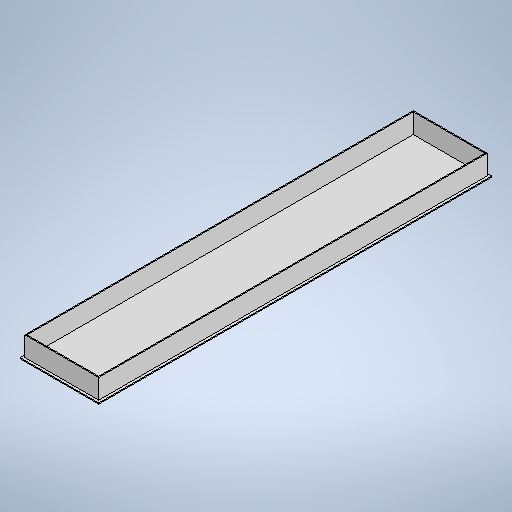
# Autodesk Inventor part: GNG НаOCl pan
Saved by Autodesk Inventor 2025 (Build 290162010, 162A)
## iProperties
Created: 2025-09-24
Part Number: GNG НаOCl pan
Material: Generic
Document SubType Name: Modeling
Designer: admin
Density: 1 g/cm^3
Appearance: Default
Mass: 50720 g
Surface Area: 102400 cm^2
Volume: 50720 cm^3
Author: admin
Autodesk Inventor part; units mm, degrees
ref_plane "YZ Plane" through (0, 0, 0) normal (1, 0, 0) x (0, 1, 0)
ref_plane "XZ Plane" through (0, 0, 0) normal (0, 1, 0) x (-1, 0, 0)
ref_plane "XY Plane" through (0, 0, 0) normal (0, 0, 1) x (1, 0, 0)
sketch "Sketch1" plane through (0, 0, 0) normal (0, 0, 1) x (1, 0, 0)
  line L0 (-400, 2000) -> (400, 2000)
  line L1 (400, 2000) -> (400, -2000)
  line L2 (400, -2000) -> (-400, -2000)
  line L3 (-400, -2000) -> (-400, 2000)
  line L4 (-400, 2000) -> (400, -2000) construction
  line L5 (400, 2000) -> (-400, -2000) construction
  point P0 (0, 0)
  dimension "d0" = 800
  dimension "d1" = 4000
  constraints: 12 end point, 2 midpoint, 2 parallel, 1 horizontal, 1 perpendicular
  measures "d0" distance of L1.end L2.end
  measures "d1" distance of L0.end L1.end
extrude "Extrusion1" add sketch "Sketch1" along normal blind 10
sketch "Sketch2" plane through (0, 0, 10) normal (0, 0, 1) x (1, 0, 0)
  line L0 (-400, -2000) -> (400, -2000) projected
  line L1 (400, -2000) -> (400, 2000) projected
  line L2 (400, 2000) -> (-400, 2000) projected
  line L3 (-400, 2000) -> (-400, -2000) projected
  line L4 (-375, -1975) -> (375, -1975)
  line L5 (375, -1975) -> (375, 1975)
  line L6 (375, 1975) -> (-375, 1975)
  line L7 (-375, 1975) -> (-375, -1975)
  line L8 (-365, -1965) -> (365, -1965)
  line L9 (365, -1965) -> (365, 1965)
  line L10 (365, 1965) -> (-365, 1965)
  line L11 (-365, 1965) -> (-365, -1965)
  point P0 (0, 0)
  dimension "d4" = 25
  dimension "d5" = 10
  constraints: 16 end point, 6 other
  measures "d4" distance between parallel lines of L3 L7
  measures "d5" distance between parallel lines of L7 L11
extrude "Extrusion2" add sketch "Sketch2" along normal blind 200 contours L7 L6 L5 L4
body "Solid1"
